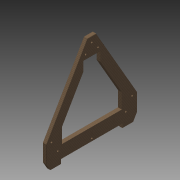
# Autodesk Inventor part: A_Frame_V2
Saved by Autodesk Inventor 2014 (Build 180170000, 170)
## iProperties
Created: 2013-12-11
Part Number: A_Frame_V2
Material: MDF Medium Density Fiberboard
Document SubType Name: Modeling
Designer: Bram
Density: 0.8 g/cm^3
Appearance: Cardboard - Corrugated
Author: Bram
Autodesk Inventor part; units mm, degrees
ref_plane "YZ Plane" through (0, 0, 0) normal (1, 0, 0) x (0, 1, 0)
ref_plane "XZ Plane" through (0, 0, 0) normal (0, 1, 0) x (-1, 0, 0)
ref_plane "XY Plane" through (0, 0, 0) normal (0, 0, 1) x (1, 0, 0)
sketch "Sketch1" plane through (0, 0, 0) normal (1, 0, 0) x (0, 1, 0)
  line L0 (216.8395, 439.9617) -> (44.7891, 141.9617)
  line L1 (117.7891, 118.7382) -> (117.7891, 178.4014)
  line L2 (117.7891, 118.7382) -> (117.7891, 108.2117)
  line L3 (117.7891, 108.2117) -> (257.2891, 108.2117)
  line L4 (44.7891, 108.2117) -> (44.7891, 141.9617)
  line L5 (44.7891, 141.9617) -> (44.7891, 61.9617)
  line L6 (217.2891, 394.9617) -> (217.2891, 350.7404)
  line L7 (217.2891, 350.7404) -> (117.7891, 178.4014)
  line L8 (217.2891, 394.9617) -> (257.2891, 394.9617)
  line L9 (297.7387, 439.9617) -> (469.7891, 141.9617)
  line L10 (297.2891, 350.7404) -> (396.7891, 178.4014)
  line L11 (396.7891, 108.2117) -> (257.2891, 108.2117)
  line L12 (396.7891, 118.7382) -> (396.7891, 178.4014)
  line L13 (396.7891, 118.7382) -> (396.7891, 108.2117)
  line L14 (469.7891, 108.2117) -> (469.7891, 141.9617)
  line L15 (469.7891, 141.9617) -> (469.7891, 61.9617)
  line L16 (297.2891, 394.9617) -> (297.2891, 350.7404)
  line L17 (297.2891, 394.9617) -> (257.2891, 394.9617)
  line L18 (216.8395, 439.9617) -> (237.0643, 474.9921)
  line L19 (297.7387, 439.9617) -> (277.5139, 474.9921)
  line L20 (237.0643, 474.9921) -> (277.5139, 474.9921)
  line L21 (44.7891, 61.9617) -> (63.3505, 29.8123)
  line L22 (63.3505, 29.8123) -> (113.3505, 29.8123)
  line L23 (113.3505, 29.8123) -> (113.3505, 49.8123)
  line L24 (113.3505, 49.8123) -> (257.2891, 49.8123)
  line L25 (469.7891, 61.9617) -> (451.2277, 29.8123)
  line L26 (451.2277, 29.8123) -> (401.2277, 29.8123)
  line L27 (401.2277, 29.8123) -> (401.2277, 49.8123)
  line L28 (401.2277, 49.8123) -> (257.2891, 49.8123)
  circle A0 centre (416.2891, 89.9617) radius 4
  circle A1 centre (445.7891, 139.9617) radius 4
  circle A2 centre (257.2891, 61.9617) radius 4
  circle A3 centre (98.2891, 89.9617) radius 4
  circle A4 centre (68.7891, 139.9617) radius 4
  circle A5 centre (286.2891, 415.9617) radius 4
  circle A6 centre (257.2891, 449.9921) radius 4
  circle A7 centre (228.2891, 415.9617) radius 4
  line L29 (117.7891, 108.2117) -> (396.7891, 108.2117)
  line L30 (396.7891, 108.2117) -> (396.7891, 178.4014)
  line L31 (396.7891, 178.4014) -> (297.2891, 350.7404)
  line L32 (297.2891, 350.7404) -> (297.2891, 394.9617)
  line L33 (297.2891, 394.9617) -> (217.2891, 394.9617)
  line L34 (217.2891, 394.9617) -> (217.2891, 350.7404)
  line L35 (217.2891, 350.7404) -> (117.7891, 178.4014)
  line L36 (117.7891, 178.4014) -> (117.7891, 108.2117)
  line L37 (237.0643, 474.9921) -> (277.5139, 474.9921)
  line L38 (277.5139, 474.9921) -> (469.7891, 141.9617)
  line L39 (469.7891, 141.9617) -> (469.7891, 61.9617)
  line L40 (469.7891, 61.9617) -> (451.2277, 29.8123)
  line L41 (451.2277, 29.8123) -> (401.2277, 29.8123)
  line L42 (401.2277, 29.8123) -> (401.2277, 49.8123)
  line L43 (401.2277, 49.8123) -> (113.3505, 49.8123)
  line L44 (113.3505, 49.8123) -> (113.3505, 29.8123)
  line L45 (113.3505, 29.8123) -> (63.3505, 29.8123)
  line L46 (63.3505, 29.8123) -> (44.7891, 61.9617)
  line L47 (44.7891, 61.9617) -> (44.7891, 141.9617)
  line L48 (44.7891, 141.9617) -> (237.0643, 474.9921)
  point P0 (0, 0)
  dimension "d29" = 29.5
  constraints: 98 end point, 8 centre point, 8 collinear, 7 perpendicular, 3 parallel, 3 point on line
extrude "Extrusion1" add sketch "Sketch1" along normal blind 18
fillet "Fillet1" radius 3 16 edges at (0, 140.9267, 308.4769) (18, 140.9267, 308.4769) (0, 44.7891, 101.9617) (18, 44.7891, 101.9617) (0, 54.0698, 45.887) (18, 54.0698, 45.887) (0, 426.2277, 29.8123) (18, 426.2277, 29.8123) (0, 460.5084, 45.887) (18, 460.5084, 45.887) (0, 469.7891, 101.9617) (18, 469.7891, 101.9617) (0, 373.6515, 308.4769) (18, 373.6515, 308.4769) (0, 257.2891, 474.9921) (18, 257.2891, 474.9921)
body "Solid1"
